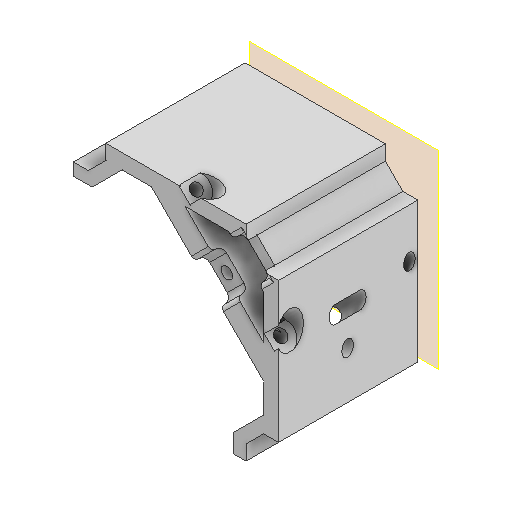
# Autodesk Inventor part: 20_Cube_Insert_Kinematic_Mirror_45_pro_v3
Saved by Autodesk Inventor 2022 (Build 260153000, 153)
## iProperties
Created: 2022-01-05
Part Number: 20_Cube_Insert_Kinematic_Mirror_45_pro_v3
Material: Generisch
Document SubType Name: Modeling
Designer: diederichbenedict
Density: 1 g/cm^3
Appearance: Vorgabe
Author: diederichbenedict
Autodesk Inventor part; units mm, degrees
ref_plane "YZ Plane" through (0, 0, 0) normal (1, 0, 0) x (0, 1, 0)
ref_plane "XZ Plane" through (0, 0, 0) normal (0, 1, 0) x (-1, 0, 0)
ref_plane "XY Plane" through (0, 0, 0) normal (0, 0, 1) x (1, 0, 0)
ref_plane "Arbeitsebene1" through (0, 0, 0) normal (0, 0, 1) x (1, 0, 0)
sketch "Skizze1" plane through (0, 0, 0) normal (0, 0, 1) x (1, 0, 0)
  line L0 (14.02, 21.9) -> (-20.02, 21.9)
  line L1 (34.79, 34.79) -> (-34.79, -34.79)
  line L2 (14.02, 21.9) -> (14.02, 14.02)
  line L3 (14.02, 14.02) -> (10.02, 10.02)
  line L4 (-20.02, 21.9) -> (-1.74, 21.9)
  line L5 (-20.02, 18.2674) -> (-24.2698, 14.02)
  line L6 (8.7191, 8.7191) -> (6.14, 6.14)
  line L7 (-20.02, 14.02) -> (-20.02, 18.2) projected
  line L8 (-20.02, 18.2) -> (14.02, 18.2) construction
  line L9 (14.02, 18.2) -> (14.02, 14.02) projected
  line L10 (14.02, 14.02) -> (18.2698, 14.02) projected
  line L11 (18.2698, 14.02) -> (18.2698, -20.02) projected
  line L12 (18.2698, -20.02) -> (14.02, -20.02) projected
  line L13 (14.02, -20.02) -> (14.02, -24.2) projected
  line L14 (14.02, -24.2) -> (-20.02, -24.2) projected
  line L15 (-20.02, -24.2) -> (-20.02, -20.02) projected
  line L16 (-20.02, -20.02) -> (-24.2698, -20.02) projected
  line L17 (-24.2698, -20.02) -> (-24.2698, 14.02) projected
  line L18 (-24.2698, 14.02) -> (-20.02, 14.02) projected
  line L19 (-23.8273, -20.7803) -> (-20.8134, -23.5239) projected
  arc A0 (-20.65, -23.8937) -> (-20.8134, -23.5239) centre (-21.15, -23.8937) ccw projected
  line L20 (-20.65, -23.8937) -> (-20.65, -26.25) projected
  arc A1 (-21.15, -26.75) -> (-20.65, -26.25) centre (-21.15, -26.25) ccw projected
  line L21 (-21.15, -26.75) -> (-26.25, -26.75) projected
  arc A2 (-26.75, -26.25) -> (-26.25, -26.75) centre (-26.25, -26.25) ccw projected
  line L22 (-26.75, -26.25) -> (-26.75, -21.15) projected
  arc A3 (-26.25, -20.65) -> (-26.75, -21.15) centre (-26.25, -21.15) ccw projected
  line L23 (-26.25, -20.65) -> (-24.1639, -20.65) projected
  arc A4 (-23.8273, -20.7803) -> (-24.1639, -20.65) centre (-24.1639, -21.15) ccw projected
  line L24 (20.75, 20.25) -> (20.75, 15.15) projected
  arc A5 (20.25, 14.65) -> (20.75, 15.15) centre (20.25, 15.15) ccw projected
  line L25 (20.25, 14.65) -> (17.8937, 14.65) projected
  arc A6 (17.5239, 14.8134) -> (17.8937, 14.65) centre (17.8937, 15.15) ccw projected
  line L26 (17.5239, 14.8134) -> (14.7803, 17.8273) projected
  arc A7 (14.65, 18.1639) -> (14.7803, 17.8273) centre (15.15, 18.1639) ccw projected
  line L27 (14.65, 18.1639) -> (14.65, 20.25) projected
  arc A8 (15.15, 20.75) -> (14.65, 20.25) centre (15.15, 20.25) ccw projected
  line L28 (15.15, 20.75) -> (20.25, 20.75) projected
  arc A9 (20.75, 20.25) -> (20.25, 20.75) centre (20.25, 20.25) ccw projected
  arc A10 (21.9, 19.9) -> (19.9, 21.9) centre (19.9, 19.9) ccw projected
  line L29 (19.9, 21.9) -> (-20.02, 21.9) projected
  line L30 (-20.02, 21.9) -> (-20.02, 18.2686) projected
  line L31 (-24.2711, 14.02) -> (-20.02, 18.2686) projected
  line L32 (-24.2711, 14.02) -> (-27.9, 14.02) projected
  line L33 (-27.9, 14.02) -> (-27.9, -25.9) projected
  arc A11 (-27.9, -25.9) -> (-25.9, -27.9) centre (-25.9, -25.9) ccw projected
  line L34 (-25.9, -27.9) -> (14.02, -27.9) projected
  line L35 (14.02, -27.9) -> (14.02, -24.2686) projected
  line L36 (18.2711, -20.02) -> (14.02, -24.2686) projected
  line L37 (18.2711, -20.02) -> (21.9, -20.02) projected
  line L38 (21.9, -20.02) -> (21.9, 19.9) projected
  line L39 (-20.02, 18.2686) -> (14.02, 18.2686)
  line L40 (-20.02, 18.2686) -> (14.02, 18.2686) construction
  line L41 (14.02, 18.2686) -> (16.1443, 16.1443)
  line L42 (16.1443, 16.1443) -> (14.02, 14.02)
  line L43 (14.02, 14.02) -> (9.7714, 18.2686)
  line L44 (-16.0848, 18.2) -> (-16.0848, 18.2686)
  line L45 (-16.0848, 18.2686) -> (-20.02, 18.2686)
  line L46 (-20.02, 18.2686) -> (-20.02, 18.2)
  line L47 (-27.9, 14.02) -> (-27.9, 11.0221)
  line L48 (-27.9, 11.0221) -> (-23.3354, 11.0221)
  line L49 (8.7191, 8.7191) -> (-0.8305, 18.2686)
  line L50 (8.7191, 8.7191) -> (22.2242, 8.7191) construction
  line L51 (4.6555, 4.6555) -> (-8.9576, 18.2686)
  line L52 (4.6555, 4.6555) -> (23.9073, 4.6555) construction
  line L53 (-16.0848, 18.2686) -> (-23.3354, 11.0221)
  line L54 (-16.0848, 18.2686) -> (-5.8338, 18.2686) construction
  line L55 (-20.02, 18.2) -> (-20.02, 21.9)
  line L56 (-24.2698, 14.02) -> (-27.9, 14.02)
  point P0 (0, 0)
  point P1 (-8.9576, 18.2686)
  point P2 (4.6555, 4.6555)
  point P3 (-24.2698, 11.0221)
  dimension "d41" = 0
  dimension "d42" = 135
  dimension "d43" = 2.9979
  dimension "d44" = 135
  dimension "d45" = 135
  dimension "d46" = 5.747
  dimension "d47" = 135.016
  constraints: 50 end point, 10 point on line, 6 horizontal, 4 equal length, 4 parallel, 3 perpendicular, 1 collinear, 1 vertical, 10 other
  measures "d41" distance between parallel lines of L39 L40
  measures "d42" angle of L39 L41
  measures "d43" distance of L47.end L47.start
  measures "d44" angle of L50 L49
  measures "d45" angle of L52 L51
  measures "d47" angle of L53 L54
extrude "Extrusion1" add sketch "Skizze1" along normal blind 33.8 contours L2 L39 L30 L0 | L41 L1 L2 | L2 L43 L39 | L46 L7 L53 L18 L5 | L39 L53 L7 L46 | L49 L1 L51 L39 | L18 L53 L48 L17 | L17 L48 L33 L32
mirror "Spiegeln1" about plane through (4.6555, 4.6555, 0) normal (0.7071068, -0.7071068, 0) of "Extrusion1"
sketch "Skizze3" plane through (16.5235, 15.7652, 0) normal (0.7071068, 0.7071068, 0) x (-0.7071068, 0.7071068, 0)
  line L0 (3.5535, 34.13) -> (-2.4465, 34.13) projected
  arc A0 (-2.4465, 34.13) -> (-2.4465, 31.13) centre (-2.4465, 32.63) ccw projected
  line L1 (-2.4465, 31.13) -> (3.5535, 31.13) projected
  arc A1 (3.5535, 31.13) -> (3.5535, 34.13) centre (3.5535, 32.63) ccw projected
  arc A2 (-16.4465, 14.05) -> (-13.4465, 14.05) centre (-14.9465, 14.05) ccw projected
  line L2 (-13.4465, 14.05) -> (-13.4465, 20.05) projected
  arc A3 (-13.4465, 20.05) -> (-16.4465, 20.05) centre (-14.9465, 20.05) ccw projected
  line L3 (-16.4465, 20.05) -> (-16.4465, 14.05) projected
  line L4 (19.5535, 29.05) -> (-11.3665, 29.05) projected
  line L5 (-11.3665, 29.05) -> (-11.3665, -1.95) projected
  line L6 (-11.3665, -1.95) -> (-15.4465, -1.95) projected
  line L7 (-18.4465, 1.05) -> (-15.4465, -1.95) projected
  line L8 (-18.4465, 1.05) -> (-18.4465, 33.05) projected
  line L9 (-15.4465, 36.05) -> (-18.4465, 33.05) projected
  line L10 (-15.4465, 36.05) -> (16.5535, 36.05) projected
  line L11 (19.5535, 33.05) -> (16.5535, 36.05) projected
  line L12 (19.5535, 33.05) -> (19.5535, 29.05) projected
  line L13 (11.5535, 33.05) -> (19.5535, 33.05) projected
  line L14 (16.5535, 36.05) -> (19.5535, 33.05) projected
  line L15 (-15.4465, 36.05) -> (16.5535, 36.05) projected
  line L16 (-18.4465, 33.05) -> (-15.4465, 36.05) projected
  line L17 (-18.4465, 1.05) -> (-18.4465, 33.05) projected
  line L18 (-15.4465, -1.95) -> (-18.4465, 1.05) projected
  line L19 (16.5535, -1.95) -> (-15.4465, -1.95) projected
  line L20 (19.5535, 1.05) -> (16.5535, -1.95) projected
  line L21 (19.5535, 29.05) -> (19.5535, 1.05) projected
  line L22 (19.5535, 29.05) -> (11.5535, 29.05) projected
  line L23 (11.5535, 29.05) -> (11.5535, 33.05) projected
  circle A4 centre (-13.4465, 31.05) radius 2 projected
  arc A5 (-16.4465, 14.05) -> (-13.4465, 14.05) centre (-14.9465, 14.05) ccw projected
  line L24 (-16.4465, 14.05) -> (-16.4465, 20.05) projected
  arc A6 (-13.4465, 20.05) -> (-16.4465, 20.05) centre (-14.9465, 20.05) ccw projected
  line L25 (-13.4465, 20.05) -> (-13.4465, 14.05) projected
  line L26 (-2.4465, 34.13) -> (3.5535, 34.13) projected
  arc A7 (3.5535, 31.13) -> (3.5535, 34.13) centre (3.5535, 32.63) ccw projected
  line L27 (3.5535, 31.13) -> (-2.4465, 31.13) projected
  arc A8 (-2.4465, 34.13) -> (-2.4465, 31.13) centre (-2.4465, 32.63) ccw projected
  circle A9 centre (-13.4465, 31.05) radius 1.45
  circle A10 centre (15.5535, 31.05) radius 1.4
  line L28 (-18.7156, 0) -> (-18.7156, 33.8) projected
  line L29 (-14.9465, 20.05) -> (-14.9465, 14.05) construction
  line L30 (-16.4465, 20.05) -> (-16.4465, 14.05)
  line L31 (-13.4465, 14.05) -> (-13.4465, 20.05)
  arc A11 (-13.4465, 20.05) -> (-16.4465, 20.05) centre (-14.9465, 20.05) ccw
  arc A12 (-16.4465, 14.05) -> (-13.4465, 14.05) centre (-14.9465, 14.05) ccw
  line L32 (3.5535, 32.63) -> (-2.4465, 32.63) construction
  line L33 (3.5535, 34.13) -> (-2.4465, 34.13)
  line L34 (-2.4465, 31.13) -> (3.5535, 31.13)
  arc A13 (3.5535, 31.13) -> (3.5535, 34.13) centre (3.5535, 32.63) ccw
  arc A14 (-2.4465, 34.13) -> (-2.4465, 31.13) centre (-2.4465, 32.63) ccw
  line L35 (-13.4465, 31.05) -> (15.5535, 31.05) construction
  line L36 (15.5535, 31.05) -> (15.5535, 2.05) construction
  line L37 (15.5535, 2.05) -> (-13.4465, 2.05) construction
  line L38 (-13.4465, 2.05) -> (-13.4465, 31.05) construction
  circle A15 centre (-13.4465, 2.05) radius 1.4
  point P0 (0.5362, 0)
  point P1 (-14.9465, 17.05)
  point P2 (0.5535, 32.63)
  dimension "d48" = 2.9
  dimension "d49" = 2.8
  dimension "d58" = 29
  dimension "d59" = 29
  dimension "d60" = 2.8
  constraints: 24 end point, 8 point on circle, 8 tangent, 7 centre point, 4 parallel, 2 coincident, 2 midpoint, 2 perpendicular, 1 concentric, 1 horizontal, 1 vertical
  measures "d48" diameter of A9
  measures "d49" diameter of A10
  measures "d58" distance of L36.end L37.end
  measures "d59" distance of L35.end L36.end
  measures "d60" diameter of A15
extrude "Extrusion2" cut sketch "Skizze3" against normal blind 33.8 contours A1 L1 A0 L0 | L3 A3 L2 A2 | A9 | A10 | A15
sketch "Skizze4" plane through (0, 0, 33.8) normal (0, 0, 1) x (1, 0, 0)
  circle A0 centre (6.675, 6.6995) radius 1.4
  line L0 (6.5855, 10.8526) -> (10.8281, 6.61) projected
  line L1 (6.5855, 10.8526) -> (2.5219, 6.7891) projected
  line L2 (6.7646, 2.5464) -> (2.5219, 6.7891) projected
  line L3 (10.8281, 6.61) -> (6.7646, 2.5464) projected
  line L4 (31.8625, 31.887) -> (-37.8747, -37.8502)
  line L5 (31.8625, 31.887) -> (-37.8747, -37.8502)
  point P0 (0, 0)
  dimension "d26" = 2.8
  constraints: 4 end point, 1 centre point, 1 point on line, 6 other
  measures "d26" diameter of A0
extrude "Extrusion3" cut sketch "Skizze4" against normal blind 20 contours A0 L4 | L4 A0
sketch "Skizze7" plane through (18.2686, 14.02, 0) normal (0.7071068, 0.7071068, 0) x (-0.7071068, 0.7071068, 0)
  circle A0 centre (-10.9784, 31.05) radius 1.45 projected
  circle A1 centre (-10.9784, 2.05) radius 1.4 projected
  point P0 (3.0042, 0)
  point P1 (18.0216, 31.05)
hole "Bohrung2" at (5.5254, 26.7632, 31.05) at (26.0315, 6.2571, 31.05) direction (-0.7071068, -0.7071068, 0) diameter 2.8 end through all counterbore diameter 6.5 counterbore depth 9
sketch "Skizze8" plane through (18.2686, -20.02, 33.8) normal (0.7073096, -0.7069039, 0) x (0, 0, -1)
  line L0 (19.75, 7.826) -> (13.75, 7.826) projected
  line L1 (13.75, 18.2308) -> (19.75, 18.2308) projected
  ellipse E0 centre (16.75, -0.0019) end of major axis (15.25, -0.0019) minor radius 1.5 projected
  circle A0 centre (16.75, 10.6717) radius 1.4
  point P0 (33.8, 1.2462)
  dimension "d61" = 2.8
  constraints: 1 centre point, 1 other
  measures "d61" diameter of A0
hole "Bohrung3" at (25.8125, -12.4718, 17.05) direction (-0.7073096, 0.7069039, 0) diameter 2.8 depth 24 tip angle 118
fillet "Rundung1" radius 1 6 edges at (3.89, 9.4846, 33.8) (9.4601, 3.9145, 33.8) (12.2855, 17.8802, 33.8) (13.6842, 18.6072, 33.8) (17.8557, 12.3101, 33.8) (18.595, 13.6965, 33.8)
